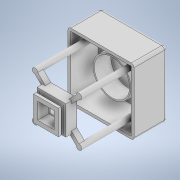
# Autodesk Inventor part: Hot Air Ballon
Saved by Autodesk Inventor 2021 (Build 250183000, 183)
## iProperties
Created: 2020-07-09
Part Number: Hot Air Ballon
Material: Generic
Document SubType Name: Modeling
Designer: saipr
Density: 1 g/cm^3
Appearance: Default
Author: saipr
Autodesk Inventor part; units mm, degrees
ref_plane "YZ Plane" through (0, 0, 0) normal (1, 0, 0) x (0, 1, 0)
ref_plane "XZ Plane" through (0, 0, 0) normal (0, 1, 0) x (-1, 0, 0)
ref_plane "XY Plane" through (0, 0, 0) normal (0, 0, 1) x (1, 0, 0)
sketch "Sketch1" plane through (0, 0, 0) normal (0, 0, 1) x (1, 0, 0)
  line L0 (38.1, -38.1) -> (-38.1, -38.1)
  line L1 (-38.1, -38.1) -> (-38.1, 38.1)
  line L2 (-38.1, 38.1) -> (38.1, 38.1)
  line L3 (38.1, 38.1) -> (38.1, -38.1)
  line L4 (38.1, -38.1) -> (-38.1, 38.1) construction
  line L5 (-38.1, -38.1) -> (38.1, 38.1) construction
  line L6 (-34.925, -34.925) -> (34.925, -34.925)
  line L7 (34.925, -34.925) -> (34.925, 34.925)
  line L8 (34.925, 34.925) -> (-34.925, 34.925)
  line L9 (-34.925, 34.925) -> (-34.925, -34.925)
  line L10 (-34.925, -34.925) -> (34.925, 34.925) construction
  line L11 (34.925, -34.925) -> (-34.925, 34.925) construction
  point P0 (0, 0)
  dimension "d0" = 76.2
  dimension "d1" = 76.2
  dimension "d2" = 69.85
  dimension "d3" = 69.85
  constraints: 24 end point, 4 midpoint, 4 parallel, 2 horizontal, 2 perpendicular
  measures "d0" distance of L1.end L2.end
  measures "d1" distance of L0.end L1.end
  measures "d2" distance of L8.end L7.end
  measures "d3" distance of L7.end L6.end
extrude "Extrusion1" add sketch "Sketch1" along normal blind 6.35 contours L0 L1 L2 L3 | L9 L8 L7 L6
extrude "Extrusion2" add sketch "Sketch1" along normal blind 38.1
fillet "Fillet1" radius 3.175 8 edges at (0, 38.1, 0) (38.1, 0, 0) (-38.1, 0, 0) (0, -38.1, 0) (38.1, 38.1, 19.05) (-38.1, 38.1, 19.05) (38.1, -38.1, 19.05) (-38.1, -38.1, 19.05)
sketch "Sketch2" plane through (0, 0, 6.35) normal (0, 0, 1) x (1, 0, 0)
  circle A0 centre (0, 0) radius 20.32
  circle A1 centre (0, 0) radius 21.9075
  dimension "d9" = 40.64
  dimension "d10" = 43.815
  constraints: 2 centre point, 2 coincident
  measures "d9" diameter of A0
  measures "d10" diameter of A1
extrude "Extrusion3" add sketch "Sketch2" along normal blind 19.05
sketch "Sketch3" plane through (0, 0, 6.35) normal (0, 0, 1) x (1, 0, 0)
  line L0 (-25.4, -25.4) -> (25.4, -25.4)
  line L1 (25.4, -25.4) -> (25.4, 25.4)
  line L2 (25.4, 25.4) -> (-25.4, 25.4)
  line L3 (-25.4, 25.4) -> (-25.4, -25.4)
  line L4 (-25.4, -25.4) -> (25.4, 25.4) construction
  line L5 (25.4, -25.4) -> (-25.4, 25.4) construction
  circle A0 centre (25.4, 25.4) radius 3.175
  circle A1 centre (-25.4, 25.4) radius 3.175
  circle A2 centre (-25.4, -25.4) radius 3.175
  circle A3 centre (25.4, -25.4) radius 3.175
  point P0 (0, 0)
  dimension "d13" = 50.8
  dimension "d14" = 50.8
  dimension "d15" = 6.35
  dimension "d16" = 6.35
  dimension "d17" = 6.35
  dimension "d18" = 6.35
  constraints: 12 end point, 4 centre point, 4 coincident, 2 midpoint, 2 parallel, 1 horizontal, 1 perpendicular
  measures "d13" distance of L2.end L1.end
  measures "d14" distance of L1.end L0.end
  measures "d15" diameter of A0
  measures "d16" diameter of A1
  measures "d17" diameter of A2
  measures "d18" diameter of A3
extrude "Extrusion4" add sketch "Sketch3" along normal blind 76.2 contours L3 A2 L0 | L0 A2 L3 | A3 L1 L0 | L0 L1 A3 | A1 L2 L3 | L3 L2 A1 | A0 L2 L1 | L1 L2 A0
sketch "Sketch4" plane through (25.4, 25.4, 82.55) normal (0, 0, 1) x (1, 0, 0)
  line L0 (0, 0) -> (-3.175, 0)
  circle A0 centre (-50.8, -50.8) radius 3.175
  circle A1 centre (0, -50.8) radius 3.175
  circle A2 centre (0, 0) radius 3.175
  circle A3 centre (-50.8, 0) radius 3.175
  circle A4 centre (-50.8, -50.8) radius 3.175 projected
  line L1 (-50.8, -47.625) -> (-47.625, -50.8)
  line L2 (1.5875, -1.5875) -> (-1.5875, 1.5875)
  circle A5 centre (-50.8, 0) radius 3.175 projected
  line L3 (-1.5875, -52.3875) -> (1.5875, -49.2125)
  line L4 (-38.862, -42.037) -> (-11.938, -42.037)
  line L5 (-8.763, -38.862) -> (-8.763, -11.938)
  line L6 (-11.938, -8.763) -> (-38.862, -8.763)
  line L7 (-42.037, -11.938) -> (-42.037, -38.862)
  line L8 (-42.037, -42.037) -> (-8.763, -8.763) construction
  line L9 (-8.763, -42.037) -> (-42.037, -8.763) construction
  line L10 (-11.0316, -39.7684) -> (-39.7684, -39.7684)
  line L11 (-39.7684, -39.7684) -> (-39.7684, -11.0316)
  line L12 (-39.7684, -11.0316) -> (-11.0316, -11.0316)
  line L13 (-11.0316, -11.0316) -> (-11.0316, -39.7684)
  line L14 (-11.0316, -39.7684) -> (-39.7684, -11.0316) construction
  line L15 (-39.7684, -39.7684) -> (-11.0316, -11.0316) construction
  line L16 (-50.8, -3.175) -> (-42.037, -11.938)
  line L17 (1.5875, -49.2125) -> (-8.763, -38.862)
  line L18 (-38.862, -8.763) -> (-47.625, 0)
  line L19 (-8.763, -11.938) -> (1.5875, -1.5875)
  line L20 (-1.5875, 1.5875) -> (-11.938, -8.763)
  line L21 (-42.037, -38.862) -> (-50.8, -47.625)
  line L22 (-47.625, -50.8) -> (-38.862, -42.037)
  line L23 (-11.938, -42.037) -> (-1.5875, -52.3875)
  line L24 (0, -50.8) -> (0, -47.625)
  line L25 (0, -3.175) -> (0, 0)
  line L26 (-50.8, -50.8) -> (-47.625, -50.8)
  line L27 (-3.175, -50.8) -> (0, -50.8)
  line L28 (-50.8, 0) -> (-50.8, -3.175)
  line L29 (-50.8, -47.625) -> (-50.8, -50.8)
  line L30 (-8.763, -11.938) -> (-8.763, -8.763)
  line L31 (-11.938, -8.763) -> (-8.763, -8.763)
  line L32 (-38.862, -8.763) -> (-42.037, -8.763)
  line L33 (-42.037, -11.938) -> (-42.037, -8.763)
  line L34 (-42.037, -38.862) -> (-42.037, -42.037)
  line L35 (-38.862, -42.037) -> (-42.037, -42.037)
  line L36 (-11.938, -42.037) -> (-8.763, -42.037)
  line L37 (-8.763, -42.037) -> (-8.763, -38.862)
  point P0 (-25.4, -25.4)
  point P1 (-25.4, -25.4)
  point P2 (-47.625, 0)
  point P3 (-3.175, -50.8)
  point P4 (0, -47.625)
  point P5 (0, -3.175)
  point P6 (-3.175, 0)
  dimension "d21" = 50.8
  dimension "d22" = 50.8
  dimension "d23" = 33.274
  dimension "d24" = 33.274
  constraints: 76 end point, 19 parallel, 10 perpendicular, 4 coincident, 4 midpoint, 4 point on circle, 3 collinear, 3 horizontal, 3 point on line, 1 vertical, 12 other
  measures "d21" distance of L0.start L28.start
  measures "d22" distance of L26.start L28.start
  measures "d23" distance of L9.end L8.end
  measures "d24" distance of L8.end L9.start
extrude "Extrusion5" add sketch "Sketch4" along normal blind 6.35
extrude "Extrusion6" add sketch "Sketch4" along normal blind 12.7 contours L31 L30 L5 L37 L36 L4 L35 L34 L7 L33 L32 L6
sketch "Sketch5" plane through (25.4, 25.4, 95.25) normal (0, 0, 1) x (1, 0, 0)
  circle A0 centre (-25.4, -25.4) radius 20.32 projected
  line L0 (-39.7495, -11.0127) -> (-11.0505, -11.0127)
  line L1 (-11.0505, -11.0127) -> (-11.0505, -39.7873)
  line L2 (-11.0505, -39.7873) -> (-39.7495, -39.7873)
  line L3 (-39.7495, -39.7873) -> (-39.7495, -11.0127)
  line L4 (-39.7495, -11.0127) -> (-11.0505, -39.7873) construction
  line L5 (-11.0505, -11.0127) -> (-39.7495, -39.7873) construction
  line L6 (-34.925, -34.925) -> (-15.875, -34.925)
  line L7 (-15.875, -34.925) -> (-15.875, -15.875)
  line L8 (-15.875, -15.875) -> (-34.925, -15.875)
  line L9 (-34.925, -15.875) -> (-34.925, -34.925)
  line L10 (-34.925, -34.925) -> (-15.875, -15.875) construction
  line L11 (-15.875, -34.925) -> (-34.925, -15.875) construction
  line L12 (-14.2875, -36.5125) -> (-36.5125, -36.5125)
  line L13 (-36.5125, -36.5125) -> (-36.5125, -14.2875)
  line L14 (-36.5125, -14.2875) -> (-14.2875, -14.2875)
  line L15 (-14.2875, -14.2875) -> (-14.2875, -36.5125)
  line L16 (-14.2875, -36.5125) -> (-36.5125, -14.2875) construction
  line L17 (-36.5125, -36.5125) -> (-14.2875, -14.2875) construction
  dimension "d29" = 19.05
  dimension "d30" = 19.05
  dimension "d33" = 22.225
  dimension "d34" = 22.225
  constraints: 36 end point, 6 midpoint, 6 parallel, 3 horizontal, 3 perpendicular, 1 point on circle
  measures "d29" distance of L8.end L7.end
  measures "d30" distance of L7.end L6.end
  measures "d33" distance of L13.end L14.end
  measures "d34" distance of L12.start L14.end
extrude "Extrusion8" add sketch "Sketch5" against normal blind 6.35 contours L1 L2 L3 L0 | L12 L13 L14 L15
extrude "Extrusion9" add sketch "Sketch5" along normal blind 6.35 contours L12 L13 L14 L15
sketch "Sketch6" plane through (25.4, 25.4, 101.6) normal (0, 0, 1) x (1, 0, 0)
  line L0 (-14.2875, -36.5125) -> (-36.5125, -36.5125) projected
  line L1 (-36.5125, -14.2875) -> (-14.2875, -14.2875)
  line L2 (-14.2875, -14.2875) -> (-14.2875, -36.5125)
  line L3 (-14.2875, -36.5125) -> (-36.5125, -36.5125)
  line L4 (-36.5125, -36.5125) -> (-36.5125, -14.2875)
  line L5 (-36.5125, -14.2875) -> (-14.2875, -36.5125) construction
  line L6 (-14.2875, -14.2875) -> (-36.5125, -36.5125) construction
  line L7 (-39.6875, -11.1125) -> (-11.1125, -11.1125)
  line L8 (-11.1125, -11.1125) -> (-11.1125, -39.6875)
  line L9 (-11.1125, -39.6875) -> (-39.6875, -39.6875)
  line L10 (-39.6875, -39.6875) -> (-39.6875, -11.1125)
  line L11 (-39.6875, -11.1125) -> (-11.1125, -39.6875) construction
  line L12 (-11.1125, -11.1125) -> (-39.6875, -39.6875) construction
  point P0 (-25.4, -25.4)
  dimension "d39" = 28.575
  dimension "d40" = 28.575
  constraints: 24 end point, 4 midpoint, 4 parallel, 2 horizontal, 2 perpendicular
  measures "d39" distance of L8.end L9.end
  measures "d40" distance of L7.end L8.end
extrude "Extrusion10" add sketch "Sketch6" against normal blind 3.175
equation "\"d34\" = d33"
body "Solid1"
